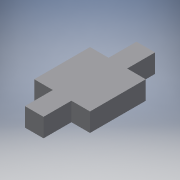
# Autodesk Inventor part: Part14
Saved by Autodesk Inventor 2018 (Build 220112000, 112)
## iProperties
Created: 2018-05-23
Part Number: Part14
Material: Generic
Document SubType Name: Modeling
Designer: lenovo
Density: 1 g/cm^3
Appearance: Default
Author: lenovo
Autodesk Inventor part; units mm, degrees
ref_plane "YZ Plane" through (0, 0, 0) normal (1, 0, 0) x (0, 1, 0)
ref_plane "XZ Plane" through (0, 0, 0) normal (0, 1, 0) x (-1, 0, 0)
ref_plane "XY Plane" through (0, 0, 0) normal (0, 0, 1) x (1, 0, 0)
sketch "Sketch1" plane through (0, 0, 0) normal (0, 1, 0) x (-1, 0, 0)
  line L0 (-25.4, 42.8625) -> (-31.75, 42.8625)
  line L1 (-31.75, 42.8625) -> (-31.75, 23.8125)
  line L2 (-31.75, 23.8125) -> (-25.4, 23.8125)
  line L3 (-25.4, 23.8125) -> (-25.4, 42.8625)
  line L4 (-25.4, 38.1) -> (-22.225, 38.1)
  line L5 (-22.225, 38.1) -> (-22.225, 28.575)
  line L6 (-22.225, 28.575) -> (-25.4, 28.575)
  line L7 (-25.4, 28.575) -> (-25.4, 38.1)
  line L8 (-31.75, 38.1) -> (-28.575, 38.1)
  line L9 (-28.575, 28.575) -> (-31.75, 28.575)
  line L10 (-31.75, 28.575) -> (-31.75, 38.1)
  line L11 (-28.575, 28.575) -> (-31.75, 28.575)
  line L12 (-31.75, 28.575) -> (-31.75, 23.8125)
  line L13 (-31.75, 23.8125) -> (-28.575, 23.8125)
  line L14 (-28.575, 23.8125) -> (-28.575, 28.575)
  line L15 (-28.575, 38.1) -> (-31.75, 38.1)
  line L16 (-31.75, 38.1) -> (-31.75, 42.8625)
  line L17 (-31.75, 42.8625) -> (-28.575, 42.8625)
  line L18 (-28.575, 42.8625) -> (-28.575, 38.1)
  point P0 (0, 0)
  dimension "d0" = 4.7625
  dimension "d1" = 4.7625
  dimension "d2" = 19.05
  dimension "d3" = 3.175
  dimension "d4" = 6.35
  constraints: 38 end point, 9 parallel, 5 horizontal, 4 perpendicular, 4 point on line
  measures "d0" distance between parallel lines of L0 L4
  measures "d1" distance between parallel lines of L2 L6
  measures "d2" distance between parallel lines of L2 L0
  measures "d3" distance between parallel lines of L5 L3
  measures "d4" distance between parallel lines of L1 L3
extrude "Extrusion2" add sketch "Sketch1" along normal blind 3.175 contours L3 L2 L14 L9 L1 L8 L18 L0 | L4 L5 L6 L3
body "Solid2"
